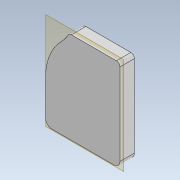
# Autodesk Inventor part: WemosCover
Saved by Autodesk Inventor 2020.2 (Build 242310000, 310)
## iProperties
Created: 2020-05-05
Part Number: WemosCover
Material: Generic
Document SubType Name: Modeling
Designer: Haashim Rehan
Density: 1 g/cm^3
Appearance: Default
Author: Haashim Rehan
Autodesk Inventor part; units mm, degrees
ref_plane "YZ Plane" through (0, 0, 0) normal (1, 0, 0) x (0, 1, 0)
ref_plane "XZ Plane" through (0, 0, 0) normal (0, 1, 0) x (-1, 0, 0)
ref_plane "XY Plane" through (0, 0, 0) normal (0, 0, 1) x (1, 0, 0)
ref_plane "Work Plane1" through (106.1845, -59.4274, 33.5479) normal (0, 0, 1) x (1, 0, 0)
sketch "Sketch2" plane through (106.1845, -59.4274, 33.5479) normal (0, 0, 1) x (1, 0, 0)
  arc A0 (-23.0626, 37.6331) -> (-14.0565, 49.6) centre (-66.1252, 79.4136) ccw
  line L0 (40, 49.6) -> (-14.0565, 49.6)
  arc A1 (-23.0626, 37.6331) -> (-40, -4.1474) centre (20, -4.1474) ccw construction
  line L1 (-40, -4.1474) -> (-40, -44.6)
  line L2 (-35, -49.6) -> (35, -49.6)
  arc A2 (-40, -44.6) -> (-35, -49.6) centre (-35, -44.6) ccw
  arc A3 (35, -49.6) -> (40, -44.6) centre (35, -44.6) ccw
  line L3 (40, -44.6) -> (40, 49.6)
  arc A4 (-23.242, 37.8072) -> (-40.25, -4.1474) centre (20, -4.1474) ccw
  arc A5 (-23.242, 37.8072) -> (-14.2017, 49.85) centre (-66.1252, 79.4136) ccw
  line L4 (-14.2017, 49.85) -> (40.25, 49.85)
  line L5 (40.25, 49.85) -> (40.25, -44.6)
  arc A6 (35, -49.85) -> (40.25, -44.6) centre (35, -44.6) ccw
  line L6 (35, -49.85) -> (-35, -49.85)
  arc A7 (-40.25, -44.6) -> (-35, -49.85) centre (-35, -44.6) ccw
  line L7 (-40.25, -44.6) -> (-40.25, -4.1474)
  arc A8 (-24.3904, 38.9214) -> (-41.85, -4.1474) centre (20, -4.1474) ccw
  arc A9 (-24.3904, 38.9214) -> (-15.1403, 51.45) centre (-66.1252, 79.4136) ccw
  line L8 (-15.1403, 51.45) -> (41.85, 51.45)
  line L9 (41.85, 51.45) -> (41.85, -44.6)
  arc A10 (35, -51.45) -> (41.85, -44.6) centre (35, -44.6) ccw
  line L10 (35, -51.45) -> (-35, -51.45)
  arc A11 (-41.85, -44.6) -> (-35, -51.45) centre (-35, -44.6) ccw
  line L11 (-41.85, -44.6) -> (-41.85, -4.1474)
  point P0 (-106.1845, 59.4274)
  dimension "d0" = 0.25
  dimension "d1" = 1.6
  constraints: 24 end point, 24 point on circle, 12 centre point, 2 horizontal, 2 vertical, 30 other
  measures "d0" radial gap between concentric circles of A1 A4
  measures "d1" radial gap between concentric circles of A4 A8
extrude "Extrusion1" add sketch "Sketch2" against normal blind 15
thicken "Thicken1" operation add thickness 1 both sides no extend neighbours yes toward (0, 0, 1) faces at (147.5012, -40.5274, 33.5479)
sketch "Sketch3" plane through (71.1845, -110.8774, 34.5479) normal (0, 0, 1) x (1, 0, 0)
  line L0 (0, 0) -> (70, 0) projected
  arc A0 (70, 0) -> (76.85, 6.85) centre (70, 6.85) ccw projected
  line L1 (76.85, 6.85) -> (76.85, 102.9) projected
  line L2 (76.85, 102.9) -> (19.8597, 102.9) projected
  arc A1 (10.6096, 90.3714) -> (19.8597, 102.9) centre (-31.1252, 130.8636) ccw projected
  arc A2 (10.6096, 90.3714) -> (-6.85, 47.3026) centre (55, 47.3026) ccw projected
  line L3 (-6.85, 47.3026) -> (-6.85, 6.85) projected
  arc A3 (-6.85, 6.85) -> (0, 0) centre (0, 6.85) ccw projected
  arc A4 (70, 1.6) -> (75.25, 6.85) centre (70, 6.85) ccw projected
  line L4 (70, 1.6) -> (0, 1.6) projected
  arc A5 (-5.25, 6.85) -> (0, 1.6) centre (0, 6.85) ccw projected
  line L5 (-5.25, 6.85) -> (-5.25, 47.3026) projected
  arc A6 (11.758, 89.2572) -> (-5.25, 47.3026) centre (55, 47.3026) ccw projected
  arc A7 (11.758, 89.2572) -> (20.7983, 101.3) centre (-31.1252, 130.8636) ccw projected
  line L6 (20.7983, 101.3) -> (75.25, 101.3) projected
  line L7 (75.25, 101.3) -> (75.25, 6.85) projected
  point P0 (-71.1845, 110.8774)
extrude "Extrusion2" add sketch "Sketch3" along normal blind 1.2 contours A3 L3 A2 A1 L2 L1 A0 L0 | L4 A5 L5 A6 A7 L6 L7 A4
fillet "Fillet1" radius 4 4 edges at (91.0442, -7.9774, 27.1479) (148.0345, -7.9774, 27.1479) (146.4345, -9.5774, 26.5479) (91.9828, -9.5774, 26.5479)
sketch "Sketch4" plane through (94.2584, -9.5774, 18.5479) normal (0, -1, 0) x (1, 0, 0)
  line L0 (0, 0) -> (0, 16) construction
  line L1 (48.1761, 0) -> (0, 0) construction
  line L2 (48.1761, 16) -> (48.1761, 0) construction
  line L3 (0, 16) -> (48.1761, 16) construction
  circle A0 centre (24.0881, 8) radius 1.875
  line L4 (0, 0) -> (0, 16) projected
  point P0 (-94.2584, -18.5479)
  point P1 (0, 8)
  point P2 (24.0881, 0)
  dimension "d11" = 3.75
  constraints: 2 midpoint, 1 centre point, 1 horizontal alignment, 1 vertical alignment
  measures "d11" diameter of A0
extrude "Extrusion3" cut sketch "Sketch4" against normal blind 1
sketch "Sketch5" plane through (146.4345, -104.0274, 18.5479) normal (-1, 0, 0) x (0, 0, 1)
  circle A0 centre (8, 45.225) radius 1.875
  line L0 (0, 0) -> (0, 90.45) construction
  line L1 (16, 0) -> (0, 0) construction
  point P0 (-18.5479, 104.0274)
  point P1 (0, 45.225)
  point P2 (8, 0)
  dimension "d15" = 3.75
  constraints: 2 midpoint, 1 centre point, 1 horizontal alignment, 1 vertical alignment
  measures "d15" diameter of A0
extrude "Extrusion4" cut sketch "Sketch5" against normal blind 1
sketch "Sketch6" plane through (71.1845, -109.2774, 18.5479) normal (0, 1, 0) x (1, 0, 0)
  circle A0 centre (35, -8) radius 1.875
  line L0 (70, -16) -> (70, 0) projected
  line L1 (0, 0) -> (70, 0) projected
  point P0 (-71.1845, 18.5479)
  point P1 (35, 0)
  point P2 (70, -8)
  dimension "d19" = 3.75
  constraints: 2 midpoint, 1 centre point, 1 horizontal alignment, 1 vertical alignment
  measures "d19" diameter of A0
sketch "Sketch7" plane through (65.9345, -104.0274, 18.5479) normal (1, 0, 0) x (0, 0, -1)
  circle A0 centre (-8, 20.2263) radius 1.875
  line L0 (-16, 40.4526) -> (0, 40.4526) projected
  line L1 (0, 40.4526) -> (0, 0) projected
  point P0 (18.5479, 104.0274)
  point P1 (-8, 40.4526)
  point P2 (0, 20.2263)
  dimension "d20" = 3.75
  constraints: 2 midpoint, 1 centre point, 1 horizontal alignment, 1 vertical alignment
  measures "d20" diameter of A0
extrude "Extrusion5" cut sketch "Sketch7" against normal blind 1
extrude "Extrusion6" cut sketch "Sketch6" against normal blind 1
fillet "Fillet4" radius 1 8 edges at (64.9345, -83.8011, 28.4229) (65.9345, -83.8011, 28.4229) (104.3095, -109.2774, 26.5479) (104.3095, -110.2774, 26.5479) (146.4345, -58.8024, 24.6729) (147.4345, -58.8024, 24.6729) (116.4715, -9.5774, 26.5479) (116.4715, -8.5774, 26.5479)
thicken "Thicken2" operation add thickness 1 both sides no extend neighbours yes toward (0, 0, 1) faces at (147.5012, -43.1941, 18.5479)
body "Solid1"
